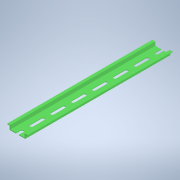
# Autodesk Inventor part: WAGO_210-112250
Saved by Autodesk Inventor 2021 (Build 250183000, 183)
## iProperties
Created: 2026-07-30
Part Number: WAGO_210-112250
Material: Generic
Catalog Web Link: www.3dfindit.com
Description: WAGO 210-112-STEEL CARRIER RAIL; 35 x 7.5 MM; 1.5 MM / 0.059 IN THICK; SLOTTED
Vendor: WAGO
Document SubType Name: Modeling
Designer: psAdmin
Manufacturer: WAGO
Mass: 11.141 g
Surface Area: 232.552 cm^2
Volume: 11.141 cm^3
Density: 1 g/cm^3
Appearance: PSOLRGB-77-178-77
Category: PARTsolutions
Company: WAGO
Title: WAGO_210-112250
Author: Cadenas PARTsolutions
Comments: STEEL CARRIER RAIL; 35 x 7.5 MM; 1.5 MM / 0.059 IN THICK; SLOTTED
PSOL_IDENT_0: {$CADENAS_DATA/23d-libs/wago/smartdesigner/0210-0112_0999-0962.prj},178 {VTYP=3D},{NB=WAGO_210-11225
PSOL_IDENT_1: 0},{LINA=WAGO_210-112250},{NN=WAGO 210-112},{DATE=08.08.2025 12:50:09},{GEOMDATE=06.04.2023 08:03:15
PSOL_IDENT_2: },{VERSION=},{LINEID=10},{WBVAR=L},{WBNUMERIC=L}  {NB=WAGO_210-112250},{LINA=WAGO_210-112250},{KT=DU
PSOL_IDENT_3: MMY},{BESTNR=210-112},{HOEHE=7.500},{L=250},{TIEFE=35.000},{FARBE=gelb chromatiert},{GEWICHT=630.000
PSOL_IDENT_4: },{EAN=4017332272292}
NB: WAGO_210-112250
NN: WAGO 210-112
NT: STEEL CARRIER RAIL; 35 x 7.5 MM; 1.5 MM / 0.059 IN THICK; SLOTTED
NBSYN: WAGO_$BESTNR.$L.
LINA: WAGO_210-112250
CATALOG: WAGO
BESTNR: 210-112
HOEHE: 7.5
L: 250
TIEFE: 35
FARBE: gelb chromatiert
GEWICHT: 630
EAN: 4017332272292
SUPPLIER: WAGO
ARTICLENO: WAGO_210-112250
BOMINFO: WAGO_210-112250
CREATOR: CADENAS GmbH
Autodesk Inventor part; units mm, degrees
ref_plane "YZ Plane" through (0, 0, 0) normal (1, 0, 0) x (0, 1, 0)
ref_plane "XZ Plane" through (0, 0, 0) normal (0, 1, 0) x (-1, 0, 0)
ref_plane "XY Plane" through (0, 0, 0) normal (0, 0, 1) x (1, 0, 0)
sketch "Skizze_1" plane through (0, 0, 0) normal (0, 0, 1) x (1, 0, 0)
  line L0 (-17.5, 0) -> (-17.5, -1)
  line L1 (-17.5, -1) -> (-13.5, -1)
  line L2 (-13.5, -1) -> (-13.5, -7.5)
  line L3 (-13.5, -7.5) -> (13.5, -7.5)
  line L4 (13.5, -7.5) -> (13.5, -1)
  line L5 (13.5, -1) -> (17.5, -1)
  line L6 (17.5, -1) -> (17.5, 0)
  line L7 (17.5, 0) -> (12.5, 0)
  line L8 (12.5, 0) -> (12.5, -6.5)
  line L9 (12.5, -6.5) -> (-12.5, -6.5)
  line L10 (-12.5, -6.5) -> (-12.5, 0)
  line L11 (-12.5, 0) -> (-17.5, 0)
  constraints: 24 end point
extrude "Extrusion1" add sketch "Skizze_1" along normal blind 250
sketch "sketch_roundrect_1" plane through (0, 0, 0) normal (0, 1, 0) x (-1, 0, 0)
  arc A0 (2.6, 9.9) -> (-2.6, 9.9) centre (0, 9.9) ccw
  line L0 (-2.6, 9.9) -> (-2.6, -9.9)
  arc A1 (-2.6, -9.9) -> (2.6, -9.9) centre (0, -9.9) ccw
  line L1 (2.6, -9.9) -> (2.6, 9.9)
  constraints: 4 end point, 4 point on circle, 2 centre point
extrude "Extrusion2" cut sketch "sketch_roundrect_1" against normal blind 50
sketch "sketch_roundrect_2" plane through (0, 0, 0) normal (0, 1, 0) x (-1, 0, 0)
  arc A0 (2.6, 45.9) -> (-2.6, 45.9) centre (0, 45.9) ccw
  line L0 (-2.6, 45.9) -> (-2.6, 26.1)
  arc A1 (-2.6, 26.1) -> (2.6, 26.1) centre (0, 26.1) ccw
  line L1 (2.6, 26.1) -> (2.6, 45.9)
  constraints: 4 end point, 4 point on circle, 2 centre point
extrude "Extrusion3" cut sketch "sketch_roundrect_2" against normal blind 50
sketch "sketch_roundrect_3" plane through (0, 0, 0) normal (0, 1, 0) x (-1, 0, 0)
  arc A0 (2.6, 81.9) -> (-2.6, 81.9) centre (0, 81.9) ccw
  line L0 (-2.6, 81.9) -> (-2.6, 62.1)
  arc A1 (-2.6, 62.1) -> (2.6, 62.1) centre (0, 62.1) ccw
  line L1 (2.6, 62.1) -> (2.6, 81.9)
  constraints: 4 end point, 4 point on circle, 2 centre point
extrude "Extrusion4" cut sketch "sketch_roundrect_3" against normal blind 50
sketch "sketch_roundrect_4" plane through (0, 0, 0) normal (0, 1, 0) x (-1, 0, 0)
  arc A0 (2.6, 117.9) -> (-2.6, 117.9) centre (0, 117.9) ccw
  line L0 (-2.6, 117.9) -> (-2.6, 98.1)
  arc A1 (-2.6, 98.1) -> (2.6, 98.1) centre (0, 98.1) ccw
  line L1 (2.6, 98.1) -> (2.6, 117.9)
  constraints: 4 end point, 4 point on circle, 2 centre point
extrude "Extrusion5" cut sketch "sketch_roundrect_4" against normal blind 50
sketch "sketch_roundrect_5" plane through (0, 0, 0) normal (0, 1, 0) x (-1, 0, 0)
  arc A0 (2.6, 153.9) -> (-2.6, 153.9) centre (0, 153.9) ccw
  line L0 (-2.6, 153.9) -> (-2.6, 134.1)
  arc A1 (-2.6, 134.1) -> (2.6, 134.1) centre (0, 134.1) ccw
  line L1 (2.6, 134.1) -> (2.6, 153.9)
  constraints: 4 end point, 4 point on circle, 2 centre point
extrude "Extrusion6" cut sketch "sketch_roundrect_5" against normal blind 50
sketch "sketch_roundrect_6" plane through (0, 0, 0) normal (0, 1, 0) x (-1, 0, 0)
  arc A0 (2.6, 189.9) -> (-2.6, 189.9) centre (0, 189.9) ccw
  line L0 (-2.6, 189.9) -> (-2.6, 170.1)
  arc A1 (-2.6, 170.1) -> (2.6, 170.1) centre (0, 170.1) ccw
  line L1 (2.6, 170.1) -> (2.6, 189.9)
  constraints: 4 end point, 4 point on circle, 2 centre point
extrude "Extrusion7" cut sketch "sketch_roundrect_6" against normal blind 50
sketch "sketch_roundrect_7" plane through (0, 0, 0) normal (0, 1, 0) x (-1, 0, 0)
  arc A0 (2.6, 225.9) -> (-2.6, 225.9) centre (0, 225.9) ccw
  line L0 (-2.6, 225.9) -> (-2.6, 206.1)
  arc A1 (-2.6, 206.1) -> (2.6, 206.1) centre (0, 206.1) ccw
  line L1 (2.6, 206.1) -> (2.6, 225.9)
  constraints: 4 end point, 4 point on circle, 2 centre point
extrude "Extrusion8" cut sketch "sketch_roundrect_7" against normal blind 50
sketch "sketch_roundrect_8" plane through (0, 0, 0) normal (0, 1, 0) x (-1, 0, 0)
  arc A0 (2.6, 261.9) -> (-2.6, 261.9) centre (0, 261.9) ccw
  line L0 (-2.6, 261.9) -> (-2.6, 242.1)
  arc A1 (-2.6, 242.1) -> (2.6, 242.1) centre (0, 242.1) ccw
  line L1 (2.6, 242.1) -> (2.6, 261.9)
  constraints: 4 end point, 4 point on circle, 2 centre point
extrude "Extrusion9" cut sketch "sketch_roundrect_8" against normal blind 50
body "Solid1"
